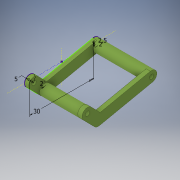
# Autodesk Inventor part: Mouth-Height-Lever
Saved by Autodesk Inventor 2018.3 (Build 223284000, 284)
## iProperties
Created: 2018-05-17
Part Number: Mouth-Height-Lever
Material: Generisch
Document SubType Name: Modeling
Designer: JochenAlt
Density: 1 g/cm^3
Appearance: Violett
Author: JochenAlt
Autodesk Inventor part; units mm, degrees
ref_plane "YZ Plane" through (0, 0, 0) normal (1, 0, 0) x (0, 1, 0)
ref_plane "XZ Plane" through (0, 0, 0) normal (0, 1, 0) x (-1, 0, 0)
ref_plane "XY Plane" through (0, 0, 0) normal (0, 0, 1) x (1, 0, 0)
sketch "Skizze1" plane through (0, 0, 0) normal (1, 0, 0) x (0, 1, 0)
  line L0 (-25.8345, 0) -> (25.2597, 0) construction
  line L1 (15, 0) -> (-15, 0) construction
  arc A0 (15.514, -2.4466) -> (14.486, 2.4466) centre (15, 0) ccw
  arc A1 (-13.2125, 1.7478) -> (-16.7875, -1.7478) centre (-15, 0) ccw
  circle A2 centre (15, 0) radius 1
  circle A3 centre (-15, 0) radius 1
  line L2 (0, 5.788) -> (0, -9.9811) construction
  line L3 (15.514, -2.4466) -> (-9.374, -7.675)
  line L4 (14.486, 2.4466) -> (-9.0595, -2.4997)
  line L5 (-11.6755, -6.9761) -> (-16.7875, -1.7478)
  line L6 (13.0082, -1.5109) -> (-7.4566, -5.8101)
  line L7 (12.5379, 0.4339) -> (-7.8087, -3.8404)
  arc A4 (14.486, 2.4466) -> (15.514, -2.4466) centre (15, 0) ccw
  circle A5 centre (-9.888, -5.2284) radius 2.5
  line L8 (-9.0595, -2.4997) -> (-13.2125, 1.7478)
  line L9 (-9.0595, -2.4997) -> (-10.402, -2.7818)
  line L10 (-9.0595, -2.4997) -> (-8.1004, -3.4806)
  point P0 (0, 0)
  dimension "d16" = 5
  dimension "d17" = 2
  dimension "d19" = 30
  dimension "d22" = 2.5
  dimension "d28" = 2
  constraints: 20 end point, 14 point on circle, 11 tangent, 6 centre point, 3 parallel, 2 coincident, 2 point on line, 1 collinear, 1 equal radius, 1 midpoint, 1 symmetric about line
  measures "d16" diameter of A1
  measures "d17" diameter of A2
  measures "d19" distance of L1.end L1.start
  measures "d22" radius of A0
  measures "d28" distance between parallel lines of L7 L6
extrude "Extrusion5" add sketch "Skizze1" along normal blind 27
ref_plane "Arbeitsebene1" through (13.5, 0, 0) normal (-1, 0, 0) x (0, 0, 1)
extrude "Extrusion6" cut sketch "Skizze1" along normal mid plane 23 from surface at 13.5 contours L3 A5 L6 A4 | A4 L7 A5 L10 L4 | L6 A5 L7 A4 | L9 A5 L5 A1 L8 | L10 A5 L9
